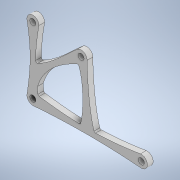
# Autodesk Inventor part: Bracket Concept MK1
Saved by Autodesk Inventor 2021 (Build 250183000, 183)
## iProperties
Created: 2021-05-11
Part Number: Bracket Concept MK1
Material: Generic
Document SubType Name: Modeling
Designer: Jawal
Density: 1 g/cm^3
Appearance: Default
Author: Jawal
Autodesk Inventor part; units mm, degrees
ref_plane "YZ Plane" through (0, 0, 0) normal (1, 0, 0) x (0, 1, 0)
ref_plane "XZ Plane" through (0, 0, 0) normal (0, 1, 0) x (-1, 0, 0)
ref_plane "XY Plane" through (0, 0, 0) normal (0, 0, 1) x (1, 0, 0)
sketch "Sketch1" plane through (0, 0, 0) normal (0, 0, 1) x (1, 0, 0)
  line L0 (-110, 70) -> (110, 70) construction
  line L1 (110, 70) -> (110, -70) construction
  line L2 (110, -70) -> (-110, -70) construction
  line L3 (-110, -70) -> (-110, 70) construction
  circle A0 centre (-90, 55) radius 5
  circle A1 centre (-90, -55) radius 5
  circle A2 centre (90, -55) radius 5
  circle A3 centre (-10, 45) radius 5
  line L4 (-67, 0) -> (-42, 0) construction
  line L5 (-42, 0) -> (-42, -30) construction
  line L6 (-42, -30) -> (-67, -30) construction
  line L7 (-67, -30) -> (-67, 0) construction
  circle A4 centre (-54.5, -11) radius 10 construction
  circle A5 centre (-63.5044, -24.4163) radius 3 construction
  circle A6 centre (-57.3559, -26.4695) radius 3 construction
  circle A7 centre (-51.263, -24.6531) radius 3 construction
  circle A8 centre (-45.3418, -26.5938) radius 3 construction
  arc A9 (-80.6122, 51.5548) -> (-99.3921, 51.5667) centre (-90, 55) ccw
  arc A10 (0, 45) -> (-16.4942, 52.6043) centre (-10, 45) ccw
  arc A11 (89.2256, -64.97) -> (88.3846, -45.1313) centre (90, -55) ccw
  line L8 (-100, 55) -> (-93.7227, 20.2343) construction
  line L9 (-93.7227, 20.2343) -> (-93.7227, 2.3339) construction
  line L10 (-93.7227, 2.3339) -> (-93.7227, -15.5707) construction
  line L11 (-93.7227, -15.5707) -> (-100, -55) construction
  spline S0 degree 4 poles (-100, 55) (-93.7227, 20.2343) (-93.7227, 2.3339) (-93.7227, -15.5707) (-100, -55) knots 1 1 1 1 1 2 2 2 2 2
  line L12 (-80, 55.0121) -> (-83.1179, 37.7603) construction
  line L13 (-33.0458, 38.469) -> (-16.4942, 52.6043) construction
  spline S1 degree 3 poles (-81.8662, -0.1941) (-57.8765, 11.5233) (-33.0458, 38.469) (-16.4942, 52.6043) knots 1.047287 1.047287 1.047287 1.047287 2 2 2 2
  line L14 (66.7614, -48.6708) -> (88.3846, -45.1313) construction
  line L15 (-90, -65) -> (-39.6885, -60.8902) construction
  line L16 (-39.6885, -60.8902) -> (0, -60.8902) construction
  line L17 (0, -60.8902) -> (36.6975, -60.8902) construction
  line L18 (36.6975, -60.8902) -> (89.2256, -64.97) construction
  spline S2 degree 4 poles (-90, -65) (-39.6885, -60.8902) (0, -60.8902) (36.6975, -60.8902) (89.2256, -64.97) knots 1 1 1 1 1 2 2 2 2 2
  spline S3 degree 3 poles (-13.6002, 30.0827) (-5.3402, 7.268) (-5.6398, -29.8026) (-10.5938, -50.667) knots 1.109736 1.109736 1.109736 1.109736 1.972131 1.972131 1.972131 1.972131
  line L19 (0, 45) -> (0, 17.1156) construction
  spline S4 degree 3 poles (0, 45) (0, 17.1156) (4.0635, -28.5965) (11.4843, -50.8799) knots 1 1 1 1 1.973632 1.973632 1.973632 1.973632
  arc A12 (-99.5185, -51.9345) -> (-88.3922, -64.8699) centre (-90, -55) ccw
  spline S5 degree 3 poles (-82.1602, -33.4696) (-73.7302, -5.1617) (-50.5606, 15.5541) (-16.7734, 31.5924) knots 1.116691 1.116691 1.116691 1.116691 1.939936 1.939936 1.939936 1.939936
  line L20 (-82.1602, -33.4696) -> (-73.7302, -5.1617) construction
  spline S6 degree 4 poles (-80, 55.0121) (-83.1179, 37.7603) (-84.6762, 24.5857) (-85.4554, 13.4176) (-85.4634, 2.054) knots 1 1 1 1 1 1.500456 1.500456 1.500456 1.500456 1.500456
  spline S7 degree 4 poles (-82.1602, -33.4696) (-82.7141, -35.9408) (-82.3572, -38.6467) (-81.9633, -41.4647) (-81.5291, -44.4067) knots 1.850189 1.850189 1.850189 1.850189 1.850189 1.936877 1.936877 1.936877 1.936877 1.936877
  line L21 (-82.1602, -33.4696) -> (-82.7141, -35.9408) construction
  spline S8 degree 4 poles (-79.5204, -46.4981) (-59.8812, -49.3583) (-42.9543, -51.1251) (-27.6277, -52.1691) (-12.9522, -52.5883) knots 1.043038 1.043038 1.043038 1.043038 1.043038 1.405573 1.405573 1.405573 1.405573 1.405573
  spline S9 degree 4 poles (13.9278, -52.5889) (30.7931, -52.1056) (47.9331, -50.8127) (66.7614, -48.6708) (88.3846, -45.1313) knots 1.574481 1.574481 1.574481 1.574481 1.574481 2 2 2 2 2
  arc A13 (-13.6002, 30.0827) -> (-16.7734, 31.5924) centre (-15.9509, 29.2316) ccw
  line L22 (-73.7302, -5.1617) -> (-50.5606, 15.5541) construction
  line L23 (-50.5606, 15.5541) -> (-16.7734, 31.5924) construction
  line L24 (-13.6002, 30.0827) -> (-5.3402, 7.268) construction
  arc A14 (-13.2443, -52.5799) -> (-10.5938, -50.667) centre (-13.0262, -50.0894) ccw
  line L25 (-5.3402, 7.268) -> (-5.6398, -29.8026) construction
  line L26 (-5.6398, -29.8026) -> (-10.5938, -50.667) construction
  line L27 (-27.6277, -52.1691) -> (-12.9522, -52.5883) construction
  arc A15 (11.4843, -50.8799) -> (13.9278, -52.5889) centre (13.8562, -50.09) ccw
  line L28 (0, 17.1156) -> (4.0635, -28.5965) construction
  line L29 (4.0635, -28.5965) -> (11.4843, -50.8799) construction
  line L30 (13.9278, -52.5889) -> (30.7931, -52.1056) construction
  line L31 (30.7931, -52.1056) -> (47.9331, -50.8127) construction
  line L32 (47.9331, -50.8127) -> (66.7614, -48.6708) construction
  arc A16 (-81.5291, -44.4067) -> (-79.5204, -46.4981) centre (-79.0558, -44.0416) ccw
  line L33 (-82.7141, -35.9408) -> (-82.3572, -38.6467) construction
  line L34 (-82.3572, -38.6467) -> (-81.9633, -41.4647) construction
  line L35 (-81.9633, -41.4647) -> (-81.5291, -44.4067) construction
  line L36 (-79.5204, -46.4981) -> (-59.8812, -49.3583) construction
  line L37 (-59.8812, -49.3583) -> (-42.9543, -51.1251) construction
  line L38 (-42.9543, -51.1251) -> (-27.6277, -52.1691) construction
  arc A17 (-85.4634, 2.054) -> (-81.8662, -0.1941) centre (-82.9634, 2.0522) ccw
  line L39 (-83.1179, 37.7603) -> (-84.6762, 24.5857) construction
  line L40 (-84.6762, 24.5857) -> (-85.4554, 13.4176) construction
  line L41 (-85.4554, 13.4176) -> (-85.4634, 2.054) construction
  line L42 (-81.8662, -0.1941) -> (-57.8765, 11.5233) construction
  line L43 (-57.8765, 11.5233) -> (-33.0458, 38.469) construction
  point P0 (0, 0)
  dimension "d1" = 70
  dimension "d2" = 70
  dimension "d3" = 110
  dimension "d4" = 110
  dimension "d5" = 10
  dimension "d6" = 10
  dimension "d7" = 10
  dimension "d8" = 10
  dimension "d9" = 55
  dimension "d10" = 55
  dimension "d11" = 55
  dimension "d12" = 180
  dimension "d13" = 90
  dimension "d14" = 90
  dimension "d15" = 10
  dimension "d16" = 45
  dimension "d17" = 42
  dimension "d18" = 30
  dimension "d19" = 0
  dimension "d20" = 25
  dimension "d21" = 20
  dimension "d22" = 6
  dimension "d23" = 6
  dimension "d24" = 6
  dimension "d25" = 11
  dimension "d26" = 12.5
  dimension "d27" = 6
  dimension "d28" = 20
  dimension "d29" = 20
  dimension "d30" = 20
  dimension "d34" = 5
  dimension "d35" = 5
  dimension "d36" = 5
  dimension "d37" = 5
  dimension "d38" = 5
  constraints: 23 point on circle, 18 centre point, 16 end point, 4 coincident, 4 parallel, 3 horizontal, 3 tangent, 3 vertical, 2 perpendicular, 42 other
  measures "d1" distance from line of point (0, 0) L2
  measures "d2" distance from line of point (0, 0) L0
  measures "d3" distance from line of L1 point (0, 0)
  measures "d4" distance from line of point (0, 0) L3
  measures "d5" diameter of A0
  measures "d6" diameter of A1
  measures "d7" diameter of A2
  measures "d8" diameter of A3
  measures "d9" vertical distance of point (0, 0) A0.centre
  measures "d10" vertical distance of point (0, 0) A1.centre
  measures "d11" vertical distance of A2.centre point (0, 0)
  measures "d12" distance of A2.centre A1.centre
  measures "d13" horizontal distance of point (0, 0) A0.centre
  measures "d14" horizontal distance of point (0, 0) A1.centre
  measures "d15" horizontal distance of point (0, 0) A3.centre
  measures "d16" vertical distance of point (0, 0) A3.centre
  measures "d17" distance from line of point (0, 0) L5
  measures "d18" distance of L4.end L5.end
  measures "d19" distance from line of L4 point (0, 0)
  measures "d20" distance of L5.end L6.end
  measures "d21" diameter of A4
  measures "d22" diameter of A5
  measures "d23" diameter of A6
  measures "d24" diameter of A7
  measures "d25" distance from line of L4 A4.centre
  measures "d26" distance from line of L7 A4.centre
  measures "d27" diameter of A8
  measures "d28" diameter of A9
  measures "d29" diameter of A10
  measures "d30" diameter of A11
  measures "d34" diameter of A13
  measures "d35" diameter of A14
  measures "d36" diameter of A15
  measures "d37" diameter of A16
  measures "d38" diameter of A17
extrude "Extrusion2" add sketch "Sketch1" along normal blind 9.5 contours S6 A17 S1 A10 S4 A15 S9 A11 S2 A12 S0 A9
equation "\"d1\" = d2"
equation "\"d4\" = d3"
equation "\"d10\" = d9"
equation "\"d11\" = d9"
equation "\"d14\" = d13"
equation "\"d26\" = 0.5 * d20"
body "Solid2"
